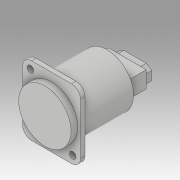
# Autodesk Inventor part: hdmi_recepticle_placeholder
Saved by Autodesk Inventor 2019.3 (Build 233278000, 278)
## iProperties
Created: 2019-06-26
Part Number: hdmi_recepticle_placeholder
Material: Generic
Document SubType Name: Modeling
Designer: Dave
Density: 1 g/cm^3
Appearance: Default
Author: Dave
Autodesk Inventor part; units mm, degrees
ref_plane "YZ Plane" through (0, 0, 0) normal (1, 0, 0) x (0, 1, 0)
ref_plane "XZ Plane" through (0, 0, 0) normal (0, 1, 0) x (-1, 0, 0)
ref_plane "XY Plane" through (0, 0, 0) normal (0, 0, 1) x (1, 0, 0)
sketch "Sketch1" plane through (0, 0, 0) normal (0, 0, 1) x (1, 0, 0)
  line L0 (4, 0) -> (22, 0)
  line L1 (26, 4) -> (26, 27)
  line L2 (22, 31) -> (4, 31)
  line L3 (0, 27) -> (0, 4)
  circle A0 centre (3.5, 27.5) radius 1.5
  circle A1 centre (22.5, 3.5) radius 1.5
  arc A2 (4, 31) -> (0, 27) centre (4, 27) ccw
  arc A3 (26, 27) -> (22, 31) centre (22, 27) ccw
  arc A4 (22, 0) -> (26, 4) centre (22, 4) ccw
  arc A5 (0, 4) -> (4, 0) centre (4, 4) ccw
  point P0 (0, 0)
  point P1 (26, 31)
  point P2 (26, 0)
  point P3 (0, 31)
  dimension "d0" = 26
  dimension "d1" = 31
  dimension "d2" = 3
  dimension "d3" = 2
  dimension "d4" = 2
  dimension "d5" = 2
  dimension "d6" = 2
  dimension "d7" = 4
  constraints: 8 end point, 8 point on circle, 8 point on line, 8 tangent, 6 centre point, 4 equal radius, 2 parallel, 1 horizontal, 1 perpendicular
  measures "d0" distance of point (26, 31) point (0, 31)
  measures "d1" distance of point (26, 0) point (26, 31)
  measures "d2" diameter of A0
  measures "d3" distance edge to line of A0 L3
  measures "d4" distance edge to line of A0 L2
  measures "d5" distance edge to line of A1 L1
  measures "d6" distance edge to line of A1 L0
  measures "d7" radius of A2
extrude "Extrusion1" add sketch "Sketch1" along normal blind 2
sketch "Sketch2" plane through (0, 0, 2) normal (0, 0, 1) x (1, 0, 0)
  circle A0 centre (13, 15.5) radius 11.75
  circle A1 centre (22.5, 3.5) radius 1.5 projected
  circle A2 centre (3.5, 27.5) radius 1.5 projected
  line L0 (22, 31) -> (4, 31) projected
  arc A3 (4, 31) -> (0, 27) centre (4, 27) ccw projected
  line L1 (0, 27) -> (0, 4) projected
  arc A4 (0, 4) -> (4, 0) centre (4, 4) ccw projected
  line L2 (4, 0) -> (22, 0) projected
  arc A5 (22, 0) -> (26, 4) centre (22, 4) ccw projected
  line L3 (26, 4) -> (26, 27) projected
  arc A6 (26, 27) -> (22, 31) centre (22, 27) ccw projected
  point P0 (0, 0)
  point P1 (0, 15.5)
  point P2 (13, 31)
  dimension "d10" = 23.5
  constraints: 2 midpoint, 1 centre point, 1 horizontal alignment, 1 vertical alignment
  measures "d10" diameter of A0
extrude "Extrusion2" add sketch "Sketch2" along normal blind 3 contours A0
sketch "Sketch3" plane through (0, 0, 0) normal (0, 0, -1) x (-1, 0, 0)
  circle A0 centre (-13, 15.5) radius 11.75 projected
  circle A1 centre (-13, 15.5) radius 11.75
  point P0 (0, 0)
  constraints: 1 centre point, 1 coincident, 1 concentric
extrude "Extrusion3" add sketch "Sketch3" along normal blind 23
sketch "Sketch4" plane through (13, 15.5, -23) normal (0, 0, -1) x (-1, 0, 0)
  line L0 (-8.5, 3.75) -> (8.5, 3.75)
  line L1 (8.5, 3.75) -> (8.5, -3.75)
  line L2 (8.5, -3.75) -> (-8.5, -3.75)
  line L3 (-8.5, -3.75) -> (-8.5, 3.75)
  circle A0 centre (0, 0) radius 11.75 projected
  point P0 (13, -15.5)
  point P1 (0, 3.75)
  point P2 (-8.5, 0)
  dimension "d15" = 17
  dimension "d16" = 7.5
  constraints: 8 end point, 2 midpoint, 2 parallel, 1 horizontal, 1 horizontal alignment, 1 perpendicular, 1 vertical alignment
  measures "d15" distance of L0.start L0.end
  measures "d16" distance of L0.end L1.end
extrude "Extrusion4" add sketch "Sketch4" along normal blind 9 contours L0 L1 L2 L3
sketch "Sketch5" plane through (13, 15.5, -32) normal (0, 0, -1) x (-1, 0, 0)
  line L0 (-7.5, 1.25) -> (-5, 2.75)
  line L1 (-5, 2.75) -> (5, 2.75)
  line L2 (5, 2.75) -> (7.5, 1.25)
  line L3 (7.5, 1.25) -> (7.5, -2.75)
  line L4 (7.5, -2.75) -> (-7.5, -2.75)
  line L5 (-7.5, -2.75) -> (-7.5, 1.25)
  line L6 (8.5, 3.75) -> (8.5, -3.75) projected
  line L7 (8.5, -3.75) -> (-8.5, -3.75) projected
  line L8 (-8.5, -3.75) -> (-8.5, 3.75) projected
  line L9 (-8.5, 3.75) -> (8.5, 3.75) projected
  circle A0 centre (0, 0) radius 11.75 projected
  point P0 (13, -15.5)
  dimension "d19" = 5.5
  dimension "d20" = 15
  dimension "d21" = 4
  dimension "d22" = 10
  dimension "d23" = 2.75
  dimension "d24" = 7.5
  constraints: 12 end point, 3 perpendicular, 2 equal length, 1 horizontal
  measures "d19" distance between parallel lines of L4 L1
  measures "d20" distance between parallel lines of L3 L5
  measures "d21" distance of L2.end L3.end
  measures "d22" distance of L0.end L1.end
  measures "d23" distance from line of A0.centre L1
  measures "d24" distance from line of A0.centre L3
extrude "Extrusion5" add sketch "Sketch5" along normal blind 3.5 contours L0 L1 L2 L3 L4 L5
body "Solid1"
